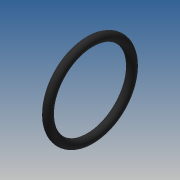
# Autodesk Inventor part: O-Ring_ra8846s
Saved by Autodesk Inventor 2021 (Build 250183000, 183)
## iProperties
Created: 2020-12-18
Part Number: O-Ring_ra8846s
Material: Gummi, Silikon
Document SubType Name: Modeling
Designer: Sander
Density: 1.25 g/cm^3
Appearance: Gummi - Schwarz
Mass: 0.0308425 g
Surface Area: 0.98696 cm^2
Volume: 0.024674 cm^3
Author: Sander
Autodesk Inventor part; units mm, degrees
ref_plane "YZ-Ebene" through (0, 0, 0) normal (1, 0, 0) x (0, 1, 0)
ref_plane "XZ-Ebene" through (0, 0, 0) normal (0, 1, 0) x (-1, 0, 0)
ref_plane "XY-Ebene" through (0, 0, 0) normal (0, 0, 1) x (1, 0, 0)
sketch "Skizze1" plane through (0, 0, 0) normal (0, 0, 1) x (1, 0, 0)
  line L0 (-0.7, 0) -> (0.7, 0) projected
  line L1 (0, -1.1) -> (0, 6.6) projected
  circle A0 centre (0, 5) radius 0.5
  point P0 (0, 0)
  dimension "d0" = 1
  dimension "d1" = 5
  constraints: 1 centre point, 1 point on line
  measures "d0" diameter of A0
  measures "d1" distance of point (0, 0) A0.centre
revolve "Umdrehung1" add sketch "Skizze1" angle 360 about axis through (-10, 0, 0) along (1, 0, 0)
